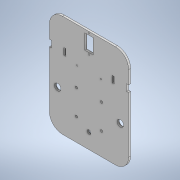
# Autodesk Inventor part: Base SD Serayu
Saved by Autodesk Inventor 2022 (Build 260153000, 153)
## iProperties
Created: 2023-12-02
Part Number: Base SD Serayu
Material: Generic
Document SubType Name: Modeling
Designer: sheva
Density: 1 g/cm^3
Appearance: Default
Author: sheva
Autodesk Inventor part; units mm, degrees
ref_plane "YZ Plane" through (0, 0, 0) normal (1, 0, 0) x (0, 1, 0)
ref_plane "XZ Plane" through (0, 0, 0) normal (0, 1, 0) x (-1, 0, 0)
ref_plane "XY Plane" through (0, 0, 0) normal (0, 0, 1) x (1, 0, 0)
sketch "Sketch1" plane through (0, 0, 0) normal (0, 0, 1) x (1, 0, 0)
  line L0 (-60, -75) -> (-60, 75)
  line L1 (-60, 75) -> (60, 75)
  line L2 (60, 75) -> (60, -75)
  ellipse E0 centre (0, 72.8464) end of major axis (0, 73.8464) minor radius 1
  line L3 (-6.15, 70.0964) -> (6.15, 70.0964)
  line L4 (6.15, 70.0964) -> (6.15, 47.3964)
  line L5 (6.15, 47.3964) -> (-6.15, 47.3964)
  line L6 (-6.15, 47.3964) -> (-6.15, 70.0964)
  circle A0 centre (0, 44.6464) radius 1
  line L7 (60, 35) -> (57, 35)
  line L8 (57, 35) -> (57, 25)
  line L9 (57, 25) -> (60, 25)
  line L10 (60, 25) -> (60, 35)
  line L11 (37.9, 35) -> (34.9, 35)
  line L12 (34.9, 35) -> (34.9, 25)
  line L13 (34.9, 25) -> (37.9, 25)
  line L14 (37.9, 25) -> (37.9, 35)
  line L15 (-60, 35) -> (-57, 35)
  line L16 (-57, 35) -> (-57, 25)
  line L17 (-57, 25) -> (-60, 25)
  line L18 (-60, 25) -> (-60, 35)
  line L19 (-37.9, 35) -> (-34.9, 35)
  line L20 (-34.9, 35) -> (-34.9, 25)
  line L21 (-34.9, 25) -> (-37.9, 25)
  line L22 (-37.9, 25) -> (-37.9, 35)
  line L23 (-0.5, 73.7124) -> (-0.5, 74.9964)
  line L24 (-0.5, 74.9964) -> (-6.15, 74.9964)
  line L25 (-6.15, 70.0964) -> (-6.15, 74.9964)
  line L26 (6.15, 70.0964) -> (-6.15, 70.0964)
  line L27 (6.15, 70.0964) -> (6.15, 74.9964)
  line L28 (6.15, 74.9964) -> (0.5, 74.9964)
  line L29 (0.5, 74.9964) -> (0.5, 73.7124)
  ellipse E1 centre (0, 72.8464) end of major axis (0, 71.8464) minor radius 1 (-0.5, 73.7124) -> (0.5, 73.7124) ccw
  line L30 (-0.5, 42.4964) -> (-0.5, 43.7803)
  ellipse E2 centre (0, 44.6464) end of major axis (0, 43.6464) minor radius 1 (0.5, 43.7803) -> (-0.5, 43.7803) ccw
  line L31 (0.5, 43.7803) -> (0.5, 42.4964)
  line L32 (6.15, 42.4964) -> (0.5, 42.4964)
  line L33 (6.15, 47.3964) -> (6.15, 42.4964)
  line L34 (-6.15, 47.3964) -> (6.15, 47.3964)
  line L35 (-6.15, 47.3964) -> (-6.15, 42.4964)
  line L36 (-0.5, 42.4964) -> (-6.15, 42.4964)
  line L37 (-6.15, 63.9464) -> (-6.15, 47.3964)
  line L38 (-6.15, 47.3964) -> (6.15, 47.3964)
  line L39 (6.15, 47.3964) -> (6.15, 63.9464)
  line L40 (6.15, 63.9464) -> (6.15, 70.0964)
  line L41 (6.15, 70.0964) -> (0, 70.0964)
  line L42 (0, 70.0964) -> (-6.15, 70.0964)
  line L43 (-6.15, 70.0964) -> (-6.15, 63.9464)
  line L44 (24.5, 3) -> (-24.5, 3)
  line L45 (-24.5, 3) -> (-24.5, 40)
  line L46 (-24.5, 40) -> (24.5, 40)
  line L47 (24.5, 40) -> (24.5, 3)
  circle A1 centre (-18, 21.5) radius 1
  circle A2 centre (18, 21.5) radius 1
  line L48 (19, -46) -> (-19, -46)
  line L49 (-19, -46) -> (-19, -8)
  line L50 (-19, -8) -> (19, -8)
  line L51 (19, -8) -> (19, -46)
  line L52 (19, -46) -> (-19, -8) construction
  line L53 (-19, -46) -> (19, -8) construction
  line L54 (22, -49) -> (-22, -49)
  line L55 (-22, -49) -> (-22, -5)
  line L56 (-22, -5) -> (22, -5)
  line L57 (22, -5) -> (22, -49)
  line L58 (22, -49) -> (-22, -5) construction
  line L59 (-22, -49) -> (22, -5) construction
  line L60 (-22, -5) -> (22, -5)
  line L61 (22, -5) -> (22, -2)
  line L62 (22, -2) -> (-22, -2)
  line L63 (-22, -2) -> (-22, -5)
  circle A3 centre (-19, -8) radius 1.75
  circle A4 centre (19, -8) radius 1.75
  circle A5 centre (-19, -46) radius 1.75
  circle A6 centre (19, -46) radius 1.75
  line L64 (-57, 65) -> (-38, 65)
  line L65 (-38, 65) -> (-38, 0.5)
  line L66 (-38, 0.5) -> (-57, 0.5)
  line L67 (-57, 0.5) -> (-57, 65)
  circle A7 centre (-47.5, -21.7) radius 5
  circle A8 centre (47.5, -21.7) radius 5
  circle A9 centre (0, -57) radius 3
  line L68 (60, -61) -> (60, -80)
  line L69 (60, -80) -> (-60, -80)
  line L70 (-60, -80) -> (-60, -62.9398)
  point P0 (0, 0)
  point P1 (-6.15, 70.0964)
  point P2 (0, -27)
  point P3 (0, -27)
  dimension "d114" = 1
  dimension "d115" = 1
  dimension "d116" = 1
  dimension "d117" = 1
  dimension "d118" = 1
  dimension "d0" = 120
  dimension "d1" = 150
  dimension "d2" = 3
  dimension "d3" = 10
  dimension "d4" = 40
  dimension "d5" = 3
  dimension "d6" = 19.1
  dimension "d7" = 3
  dimension "d8" = 10
  dimension "d9" = 3
  dimension "d10" = 19.1
  dimension "d94" = 49
  dimension "d95" = 37
  dimension "d96" = 32.5036
  dimension "d98" = 35
  dimension "d99" = 2
  dimension "d100" = 2
  dimension "d101" = 36
  dimension "d102" = 6.5
  dimension "d103" = 6.5
  dimension "d104" = 18.5
  dimension "d105" = 18.5
  dimension "d113" = 72
  dimension "d119" = 90
  dimension "d120" = 90
  dimension "d121" = 90
  dimension "d122" = 90
  dimension "d123" = 90
  dimension "d124" = 90
  dimension "d125" = 90
  dimension "d126" = 90
  dimension "d127" = 90
  dimension "d128" = 90
  dimension "d129" = 35.5
  dimension "d130" = 53.85
  dimension "d131" = 53.85
  dimension "d132" = 59.5
  dimension "d133" = 59.5
  dimension "d134" = 60.5
  dimension "d135" = 66.15
  dimension "d136" = 66.15
  dimension "d137" = 94.9
  dimension "d138" = 0
  dimension "d139" = 10
  dimension "d140" = 39.9964
  dimension "d141" = 35.0964
  dimension "d142" = 12.3964
  dimension "d143" = 35.0964
  dimension "d145" = 39.9964
  dimension "d146" = 7.4964
  dimension "d147" = 12.3964
  dimension "d148" = 0
  dimension "d149" = 60
  dimension "d150" = 35
  dimension "d151" = 70.0964
  dimension "d152" = 6.15
  dimension "d153" = 6.15
  dimension "d154" = 6.15
  dimension "d155" = 0.5
  dimension "d156" = 70.0964
  dimension "d157" = 6.15
  dimension "d158" = 47.3964
  dimension "d159" = 6.15
  dimension "d160" = 6.15
  constraints: 142 end point, 35 parallel, 10 centre point, 9 horizontal, 9 perpendicular, 5 midpoint, 5 point on line, 4 coincident, 4 vertical, 1 equal radius, 1 tangent, 12 other
  measures "d0" distance of L1.start L1.end
  measures "d1" distance of L0.start L0.end
  measures "d2" distance of L9.end L8.end
  measures "d3" distance of L8.end L7.end
  measures "d4" distance between parallel lines of L1 L7
  measures "d5" distance of L13.end L12.end
  measures "d6" distance between parallel lines of L8 L14
  measures "d7" distance of L16.end L17.end
  measures "d8" distance of L15.end L16.end
  measures "d9" distance of L20.end L21.end
  measures "d10" distance between parallel lines of L22 L16
  measures "d94" distance of L45.end L46.end
  measures "d95" distance of L44.end L45.end
  measures "d96" distance between parallel lines of L1 L32
  measures "d98" distance between parallel lines of L1 L46
  measures "d99" diameter of A1
  measures "d100" diameter of A2
  measures "d101" distance of A2.centre A1.centre
  measures "d102" distance from line of L45 A1.centre
  measures "d103" distance from line of L47 A2.centre
  measures "d104" distance from line of L46 A2.centre
  measures "d105" distance from line of L46 A1.centre
  measures "d113" distance between parallel lines of L44 L1
  measures "d119" angle of L2 L41
  measures "d120" angle of L2 L3
  measures "d121" angle of L2 L34
  measures "d122" angle of L7 L27
  measures "d123" angle of L7 L4
  measures "d124" angle of L7 L33
  measures "d125" angle of L7 L23
  measures "d126" angle of L7 L25
  measures "d127" angle of L7 L35
  measures "d128" angle of L7 L6
  measures "d129" distance between parallel lines of L2 L47
  measures "d130" distance between parallel lines of L2 L40
  measures "d131" distance between parallel lines of L2 L39
  measures "d132" distance between parallel lines of L2 L29
  measures "d133" distance between parallel lines of L2 L31
  measures "d134" distance between parallel lines of L2 L30
  measures "d135" distance between parallel lines of L2 L43
  measures "d136" distance between parallel lines of L2 L37
  measures "d137" distance between parallel lines of L2 L20
  measures "d138" distance between parallel lines of L7 L11
  measures "d139" distance between parallel lines of L7 L13
  measures "d140" distance between parallel lines of L7 L28
  measures "d141" distance between parallel lines of L7 L26
  measures "d142" distance between parallel lines of L7 L5
  measures "d143" distance between parallel lines of L42 L7
  measures "d145" distance between parallel lines of L7 L24
  measures "d146" distance between parallel lines of L7 L36
  measures "d147" distance between parallel lines of L38 L7
  measures "d148" distance between parallel lines of L7 L19
  measures "d149" distance from line of point (0, 0) L2
  measures "d150" distance from line of point (0, 0) L7
  measures "d151" distance from line of point (0, 0) L41
  measures "d152" distance from line of point (0, 0) L27
  measures "d153" distance from line of point (0, 0) L4
  measures "d154" distance from line of point (0, 0) L33
  measures "d155" distance from line of point (0, 0) L23
  measures "d156" distance from line of point (0, 0) L3
  measures "d157" distance from line of point (0, 0) L25
  measures "d158" distance from line of point (0, 0) L34
  measures "d159" distance from line of point (0, 0) L35
  measures "d160" distance from line of point (0, 0) L6
extrude "Extrusion1" add sketch "Sketch1" along normal blind 3 contours L0 L17 L67 L66 L65 L64 L15 L1 L2 L7 L8 L9 L68 L69 L70 | L16 L67 L64 L65 L66 | E0 L29 L28 L27 L3 L25 L24 L23 | L5 L33 L32 L31 A0 L30 L36 L35 | L44 L45 L46 L47 | A5 L49 A3 L50 A4 L51 A6 L48 | L54 L55 L56 L57 | L56 L63 L62 L61
fillet "Fillet1" radius 20 4 edges at (-60, 75, 1.5) (60, 75, 1.5) (-60, -80, 1.5) (60, -80, 1.5)
body "Solid1"
